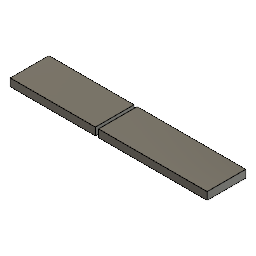
Untitled (Autodesk Fusion 360 design; units mm, degrees)
Autodesk Fusion 360 part; units mm, degrees
box "BoxPrimitive1" add length 50 width 110 height 10 placed x (0, 0, -1) y (-1, 0, 0) z (0, 1, 0) at (160, 0, 60) makes body 1
box "BoxPrimitive1'" add length 50 width 140 height 10 placed x (0, 0, -1) y (-1, 0, 0) z (0, 1, 0) at (350, 0, 50) separate body makes body 2 in component "Component"
component "Component" placed x (-1, 0, 0) y (0, -1, 0) z (0, 0, 1) at (514, 10, 10)
